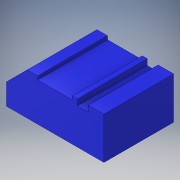
# Autodesk Inventor part: lift holder
Saved by Autodesk Inventor 2019 (Build 230136000, 136)
## iProperties
Created: 2018-10-20
Part Number: lift holder
Material: PC/ABS Plastic
Document SubType Name: Modeling
Designer: User
Density: 0.357273 g/cm^3
Appearance: Blue - Wall Paint - Glossy
Author: User
Autodesk Inventor part; units mm, degrees
ref_plane "YZ Plane" through (0, 0, 0) normal (1, 0, 0) x (0, 1, 0)
ref_plane "XZ Plane" through (0, 0, 0) normal (0, 1, 0) x (-1, 0, 0)
ref_plane "XY Plane" through (0, 0, 0) normal (0, 0, 1) x (1, 0, 0)
sketch "Sketch1" plane through (0, 0, 0) normal (0, 1, 0) x (-1, 0, 0)
  line L0 (0, 0) -> (88.9, 0)
  line L1 (88.9, 0) -> (88.9, -63.5)
  line L2 (88.9, -63.5) -> (0, -63.5)
  line L3 (0, -63.5) -> (0, 0)
  dimension "d0" = 88.9
  dimension "d1" = 63.5
  constraints: 8 end point, 2 parallel, 1 horizontal, 1 perpendicular
  measures "d0" distance of L1.end L2.end
  measures "d1" distance of L0.end L1.end
extrude "Extrusion1" add sketch "Sketch1" along normal blind 38.1
sketch "Sketch2" plane through (0, 38.1, 0) normal (0, 1, 0) x (1, 0, 0)
  line L0 (0, 63.5) -> (-88.9, 63.5) projected
  line L1 (-88.9, 0) -> (0, 0) projected
  line L2 (-28.575, 63.5) -> (-60.325, 63.5)
  line L3 (-60.325, 63.5) -> (-60.325, 0)
  line L4 (-60.325, 0) -> (-28.575, 0)
  line L5 (-28.575, 0) -> (-28.575, 63.5)
  line L6 (0, 0) -> (0, 63.5) projected
  dimension "d4" = 88.9
  dimension "d5" = 31.75
  dimension "d6" = 28.575
  constraints: 8 end point, 2 parallel, 2 point on line, 1 horizontal, 1 perpendicular
  measures "d4" distance of L1.start L1.end
  measures "d5" distance between parallel lines of L5 L3
  measures "d6" distance between parallel lines of L6 L5
extrude "Extrusion2" cut sketch "Sketch2" against normal blind 3.175 contours L5 L1 L3 L0
chamfer "Chamfer1" distance 19.05 angle 45 1 edges at (-88.9, 38.1, -31.75)
sketch "Sketch3" plane through (0, 38.1, 0) normal (0, 1, 0) x (1, 0, 0)
  line L0 (-28.575, 63.5) -> (-28.575, 0) projected
  line L1 (-28.575, 0) -> (0, 0) projected
  line L2 (0, 0) -> (0, 63.5) projected
  line L3 (0, 63.5) -> (-28.575, 63.5) projected
  line L4 (-88.9, 63.5) -> (0, 63.5) projected
  line L5 (0, 0) -> (-88.9, 0) projected
  line L6 (-24.003, 63.5) -> (-14.097, 63.5)
  line L7 (-14.097, 63.5) -> (-14.097, 0)
  line L8 (-14.097, 0) -> (-24.003, 0)
  line L9 (-24.003, 0) -> (-24.003, 63.5)
  dimension "d13" = 4.572
  dimension "d14" = 9.906
  constraints: 8 end point, 2 parallel, 2 point on line, 1 horizontal, 1 perpendicular
  measures "d13" distance between parallel lines of L0 L9
  measures "d14" distance between parallel lines of L9 L7
extrude "Extrusion3" cut sketch "Sketch3" against normal blind 5.461 contours L3 L7 L1 L9
equation "\"d6\" = -0.5 * d5 + 0.5 * d4"
body "Solid1"
